Autodesk Inventor part; units mm, degrees
(part 10 of 12)
  line L8077 (-17.2005, 26.4334) -> (-16.2005, 26.4334)
  line L8078 (-16.2005, 26.4334) -> (-16.2005, 25.4334)
  line L8079 (-16.7593, 25.4334) -> (-17.7593, 25.4334)
  line L8080 (-17.7593, 25.4334) -> (-17.7593, 26.4334)
  line L8081 (-17.7593, 26.4334) -> (-16.7593, 26.4334)
  line L8082 (-16.7593, 26.4334) -> (-16.7593, 25.4334)
  line L8083 (-17.4197, 25.4334) -> (-18.4197, 25.4334)
  line L8084 (-18.4197, 25.4334) -> (-18.4197, 26.4334)
  line L8085 (-18.4197, 26.4334) -> (-17.4197, 26.4334)
  line L8086 (-17.4197, 26.4334) -> (-17.4197, 25.4334)
  line L8087 (-18.0166, 25.4334) -> (-19.0166, 25.4334)
  line L8088 (-19.0166, 25.4334) -> (-19.0166, 26.4334)
  line L8089 (-19.0166, 26.4334) -> (-18.0166, 26.4334)
  line L8090 (-18.0166, 26.4334) -> (-18.0166, 25.4334)
  line L8091 (-18.6643, 25.4334) -> (-19.6643, 25.4334)
  line L8092 (-19.6643, 25.4334) -> (-19.6643, 26.4334)
  line L8093 (-19.6643, 26.4334) -> (-18.6643, 26.4334)
  line L8094 (-18.6643, 26.4334) -> (-18.6643, 25.4334)
  line L8095 (-19.2739, 25.4334) -> (-20.2739, 25.4334)
  line L8096 (-20.2739, 25.4334) -> (-20.2739, 26.4334)
  line L8097 (-20.2739, 26.4334) -> (-19.2739, 26.4334)
  line L8098 (-19.2739, 26.4334) -> (-19.2739, 25.4334)
  line L8099 (-19.6676, 25.4334) -> (-20.6676, 25.4334)
  line L8100 (-20.6676, 25.4334) -> (-20.6676, 26.4334)
  line L8101 (-20.6676, 26.4334) -> (-19.6676, 26.4334)
  line L8102 (-19.6676, 26.4334) -> (-19.6676, 25.4334)
  line L8103 (-20.0867, 25.4334) -> (-21.0867, 25.4334)
  line L8104 (-21.0867, 25.4334) -> (-21.0867, 26.4334)
  line L8105 (-21.0867, 26.4334) -> (-20.0867, 26.4334)
  line L8106 (-20.0867, 26.4334) -> (-20.0867, 25.4334)
  line L8107 (-20.4931, 25.4334) -> (-21.4931, 25.4334)
  line L8108 (-21.4931, 25.4334) -> (-21.4931, 26.4334)
  line L8109 (-21.4931, 26.4334) -> (-20.4931, 26.4334)
  line L8110 (-20.4931, 26.4334) -> (-20.4931, 25.4334)
  line L8111 (-21.1916, 25.4334) -> (-22.1916, 25.4334)
  line L8112 (-22.1916, 25.4334) -> (-22.1916, 26.4334)
  line L8113 (-22.1916, 26.4334) -> (-21.1916, 26.4334)
  line L8114 (-21.1916, 26.4334) -> (-21.1916, 25.4334)
  line L8115 (-21.8393, 25.4334) -> (-22.8393, 25.4334)
  line L8116 (-22.8393, 25.4334) -> (-22.8393, 26.4334)
  line L8117 (-22.8393, 26.4334) -> (-21.8393, 26.4334)
  line L8118 (-21.8393, 26.4334) -> (-21.8393, 25.4334)
  line L8119 (-13.0255, 25.4588) -> (-14.0255, 25.4588)
  line L8120 (-14.0255, 25.4588) -> (-14.0255, 26.4588)
  line L8121 (-14.0255, 26.4588) -> (-13.0255, 26.4588)
  line L8122 (-13.0255, 26.4588) -> (-13.0255, 25.4588)
  line L8123 (-14.74, 25.4588) -> (-15.74, 25.4588)
  line L8124 (-15.74, 25.4588) -> (-15.74, 26.4588)
  line L8125 (-15.74, 26.4588) -> (-14.74, 26.4588)
  line L8126 (-14.74, 26.4588) -> (-14.74, 25.4588)
  line L8127 (-15.5147, 25.4588) -> (-16.5147, 25.4588)
  line L8128 (-16.5147, 25.4588) -> (-16.5147, 26.4588)
  line L8129 (-16.5147, 26.4588) -> (-15.5147, 26.4588)
  line L8130 (-15.5147, 26.4588) -> (-15.5147, 25.4588)
  line L8131 (-16.1878, 25.4588) -> (-17.1878, 25.4588)
  line L8132 (-17.1878, 25.4588) -> (-17.1878, 26.4588)
  line L8133 (-17.1878, 26.4588) -> (-16.1878, 26.4588)
  line L8134 (-16.1878, 26.4588) -> (-16.1878, 25.4588)
  line L8135 (-16.7847, 25.4588) -> (-17.7847, 25.4588)
  line L8136 (-17.7847, 25.4588) -> (-17.7847, 26.4588)
  line L8137 (-17.7847, 26.4588) -> (-16.7847, 26.4588)
  line L8138 (-16.7847, 26.4588) -> (-16.7847, 25.4588)
  line L8139 (-17.4197, 25.4588) -> (-18.4197, 25.4588)
  line L8140 (-18.4197, 25.4588) -> (-18.4197, 26.4588)
  line L8141 (-18.4197, 26.4588) -> (-17.4197, 26.4588)
  line L8142 (-17.4197, 26.4588) -> (-17.4197, 25.4588)
  line L8143 (-18.3341, 25.4588) -> (-19.3341, 25.4588)
  line L8144 (-19.3341, 25.4588) -> (-19.3341, 26.4588)
  line L8145 (-19.3341, 26.4588) -> (-18.3341, 26.4588)
  line L8146 (-18.3341, 26.4588) -> (-18.3341, 25.4588)
  line L8147 (-19.2739, 25.4588) -> (-20.2739, 25.4588)
  line L8148 (-20.2739, 25.4588) -> (-20.2739, 26.4588)
  line L8149 (-20.2739, 26.4588) -> (-19.2739, 26.4588)
  line L8150 (-19.2739, 26.4588) -> (-19.2739, 25.4588)
  line L8151 (-19.6676, 25.4588) -> (-20.6676, 25.4588)
  line L8152 (-20.6676, 25.4588) -> (-20.6676, 26.4588)
  line L8153 (-20.6676, 26.4588) -> (-19.6676, 26.4588)
  line L8154 (-19.6676, 26.4588) -> (-19.6676, 25.4588)
  line L8155 (-20.0867, 25.4588) -> (-21.0867, 25.4588)
  line L8156 (-21.0867, 25.4588) -> (-21.0867, 26.4588)
  line L8157 (-21.0867, 26.4588) -> (-20.0867, 26.4588)
  line L8158 (-20.0867, 26.4588) -> (-20.0867, 25.4588)
  line L8159 (-20.4931, 25.4588) -> (-21.4931, 25.4588)
  line L8160 (-21.4931, 25.4588) -> (-21.4931, 26.4588)
  line L8161 (-21.4931, 26.4588) -> (-20.4931, 26.4588)
  line L8162 (-20.4931, 26.4588) -> (-20.4931, 25.4588)
  line L8163 (-21.1916, 25.4588) -> (-22.1916, 25.4588)
  line L8164 (-22.1916, 25.4588) -> (-22.1916, 26.4588)
  line L8165 (-22.1916, 26.4588) -> (-21.1916, 26.4588)
  line L8166 (-21.1916, 26.4588) -> (-21.1916, 25.4588)
  line L8167 (-21.852, 25.4588) -> (-22.852, 25.4588)
  line L8168 (-22.852, 25.4588) -> (-22.852, 26.4588)
  line L8169 (-22.852, 26.4588) -> (-21.852, 26.4588)
  line L8170 (-21.852, 26.4588) -> (-21.852, 25.4588)
  line L8171 (-12.4667, 25.4842) -> (-13.4667, 25.4842)
  line L8172 (-13.4667, 25.4842) -> (-13.4667, 26.4842)
  line L8173 (-13.4667, 26.4842) -> (-12.4667, 26.4842)
  line L8174 (-12.4667, 26.4842) -> (-12.4667, 25.4842)
  line L8175 (-13.0509, 25.4842) -> (-14.0509, 25.4842)
  line L8176 (-14.0509, 25.4842) -> (-14.0509, 26.4842)
  line L8177 (-14.0509, 26.4842) -> (-13.0509, 26.4842)
  line L8178 (-13.0509, 26.4842) -> (-13.0509, 25.4842)
  line L8179 (-14.7654, 25.4842) -> (-15.7654, 25.4842)
  line L8180 (-15.7654, 25.4842) -> (-15.7654, 26.4842)
  line L8181 (-15.7654, 26.4842) -> (-14.7654, 26.4842)
  line L8182 (-14.7654, 26.4842) -> (-14.7654, 25.4842)
  line L8183 (-15.5528, 25.4842) -> (-16.5528, 25.4842)
  line L8184 (-16.5528, 25.4842) -> (-16.5528, 26.4842)
  line L8185 (-16.5528, 26.4842) -> (-15.5528, 26.4842)
  line L8186 (-15.5528, 26.4842) -> (-15.5528, 25.4842)
  line L8187 (-16.1497, 25.4842) -> (-17.1497, 25.4842)
  line L8188 (-17.1497, 25.4842) -> (-17.1497, 26.4842)
  line L8189 (-17.1497, 26.4842) -> (-16.1497, 26.4842)
  line L8190 (-16.1497, 26.4842) -> (-16.1497, 25.4842)
  line L8191 (-16.7974, 25.4842) -> (-17.7974, 25.4842)
  line L8192 (-17.7974, 25.4842) -> (-17.7974, 26.4842)
  line L8193 (-17.7974, 26.4842) -> (-16.7974, 26.4842)
  line L8194 (-16.7974, 26.4842) -> (-16.7974, 25.4842)
  line L8195 (-17.3943, 25.4842) -> (-18.3943, 25.4842)
  line L8196 (-18.3943, 25.4842) -> (-18.3943, 26.4842)
  line L8197 (-18.3943, 26.4842) -> (-17.3943, 26.4842)
  line L8198 (-17.3943, 26.4842) -> (-17.3943, 25.4842)
  line L8199 (-18.3341, 25.4842) -> (-19.3341, 25.4842)
  line L8200 (-19.3341, 25.4842) -> (-19.3341, 26.4842)
  line L8201 (-19.3341, 26.4842) -> (-18.3341, 26.4842)
  line L8202 (-18.3341, 26.4842) -> (-18.3341, 25.4842)
  line L8203 (-19.2739, 25.4842) -> (-20.2739, 25.4842)
  line L8204 (-20.2739, 25.4842) -> (-20.2739, 26.4842)
  line L8205 (-20.2739, 26.4842) -> (-19.2739, 26.4842)
  line L8206 (-19.2739, 26.4842) -> (-19.2739, 25.4842)
  line L8207 (-19.6676, 25.4842) -> (-20.6676, 25.4842)
  line L8208 (-20.6676, 25.4842) -> (-20.6676, 26.4842)
  line L8209 (-20.6676, 26.4842) -> (-19.6676, 26.4842)
  line L8210 (-19.6676, 26.4842) -> (-19.6676, 25.4842)
  line L8211 (-20.1121, 25.4842) -> (-21.1121, 25.4842)
  line L8212 (-21.1121, 25.4842) -> (-21.1121, 26.4842)
  line L8213 (-21.1121, 26.4842) -> (-20.1121, 26.4842)
  line L8214 (-20.1121, 26.4842) -> (-20.1121, 25.4842)
  line L8215 (-20.4931, 25.4842) -> (-21.4931, 25.4842)
  line L8216 (-21.4931, 25.4842) -> (-21.4931, 26.4842)
  line L8217 (-21.4931, 26.4842) -> (-20.4931, 26.4842)
  line L8218 (-20.4931, 26.4842) -> (-20.4931, 25.4842)
  line L8219 (-21.1789, 25.4842) -> (-22.1789, 25.4842)
  line L8220 (-22.1789, 25.4842) -> (-22.1789, 26.4842)
  line L8221 (-22.1789, 26.4842) -> (-21.1789, 26.4842)
  line L8222 (-21.1789, 26.4842) -> (-21.1789, 25.4842)
  line L8223 (-21.8647, 25.4842) -> (-22.8647, 25.4842)
  line L8224 (-22.8647, 25.4842) -> (-22.8647, 26.4842)
  line L8225 (-22.8647, 26.4842) -> (-21.8647, 26.4842)
  line L8226 (-21.8647, 26.4842) -> (-21.8647, 25.4842)
  line L8227 (-12.4921, 25.5096) -> (-13.4921, 25.5096)
  line L8228 (-13.4921, 25.5096) -> (-13.4921, 26.5096)
  line L8229 (-13.4921, 26.5096) -> (-12.4921, 26.5096)
  line L8230 (-12.4921, 26.5096) -> (-12.4921, 25.5096)
  line L8231 (-13.0763, 25.5096) -> (-14.0763, 25.5096)
  line L8232 (-14.0763, 25.5096) -> (-14.0763, 26.5096)
  line L8233 (-14.0763, 26.5096) -> (-13.0763, 26.5096)
  line L8234 (-13.0763, 26.5096) -> (-13.0763, 25.5096)
  line L8235 (-14.7908, 25.5096) -> (-15.7908, 25.5096)
  line L8236 (-15.7908, 25.5096) -> (-15.7908, 26.5096)
  line L8237 (-15.7908, 26.5096) -> (-14.7908, 26.5096)
  line L8238 (-14.7908, 26.5096) -> (-14.7908, 25.5096)
  line L8239 (-15.8576, 25.5096) -> (-16.8576, 25.5096)
  line L8240 (-16.8576, 25.5096) -> (-16.8576, 26.5096)
  line L8241 (-16.8576, 26.5096) -> (-15.8576, 26.5096)
  line L8242 (-15.8576, 26.5096) -> (-15.8576, 25.5096)
  line L8243 (-16.8228, 25.5096) -> (-17.8228, 25.5096)
  line L8244 (-17.8228, 25.5096) -> (-17.8228, 26.5096)
  line L8245 (-17.8228, 26.5096) -> (-16.8228, 26.5096)
  line L8246 (-16.8228, 26.5096) -> (-16.8228, 25.5096)
  line L8247 (-17.3943, 25.5096) -> (-18.3943, 25.5096)
  line L8248 (-18.3943, 25.5096) -> (-18.3943, 26.5096)
  line L8249 (-18.3943, 26.5096) -> (-17.3943, 26.5096)
  line L8250 (-17.3943, 26.5096) -> (-17.3943, 25.5096)
  line L8251 (-18.3341, 25.5096) -> (-19.3341, 25.5096)
  line L8252 (-19.3341, 25.5096) -> (-19.3341, 26.5096)
  line L8253 (-19.3341, 26.5096) -> (-18.3341, 26.5096)
  line L8254 (-18.3341, 26.5096) -> (-18.3341, 25.5096)
  line L8255 (-19.2739, 25.5096) -> (-20.2739, 25.5096)
  line L8256 (-20.2739, 25.5096) -> (-20.2739, 26.5096)
  line L8257 (-20.2739, 26.5096) -> (-19.2739, 26.5096)
  line L8258 (-19.2739, 26.5096) -> (-19.2739, 25.5096)
  line L8259 (-19.6676, 25.5096) -> (-20.6676, 25.5096)
  line L8260 (-20.6676, 25.5096) -> (-20.6676, 26.5096)
  line L8261 (-20.6676, 26.5096) -> (-19.6676, 26.5096)
  line L8262 (-19.6676, 26.5096) -> (-19.6676, 25.5096)
  line L8263 (-20.1121, 25.5096) -> (-21.1121, 25.5096)
  line L8264 (-21.1121, 25.5096) -> (-21.1121, 26.5096)
  line L8265 (-21.1121, 26.5096) -> (-20.1121, 26.5096)
  line L8266 (-20.1121, 26.5096) -> (-20.1121, 25.5096)
  line L8267 (-20.4931, 25.5096) -> (-21.4931, 25.5096)
  line L8268 (-21.4931, 25.5096) -> (-21.4931, 26.5096)
  line L8269 (-21.4931, 26.5096) -> (-20.4931, 26.5096)
  line L8270 (-20.4931, 26.5096) -> (-20.4931, 25.5096)
  line L8271 (-21.1789, 25.5096) -> (-22.1789, 25.5096)
  line L8272 (-22.1789, 25.5096) -> (-22.1789, 26.5096)
  line L8273 (-22.1789, 26.5096) -> (-21.1789, 26.5096)
  line L8274 (-21.1789, 26.5096) -> (-21.1789, 25.5096)
  line L8275 (-21.8774, 25.5096) -> (-22.8774, 25.5096)
  line L8276 (-22.8774, 25.5096) -> (-22.8774, 26.5096)
  line L8277 (-22.8774, 26.5096) -> (-21.8774, 26.5096)
  line L8278 (-21.8774, 26.5096) -> (-21.8774, 25.5096)
  line L8279 (-12.5175, 25.535) -> (-13.5175, 25.535)
  line L8280 (-13.5175, 25.535) -> (-13.5175, 26.535)
  line L8281 (-13.5175, 26.535) -> (-12.5175, 26.535)
  line L8282 (-12.5175, 26.535) -> (-12.5175, 25.535)
  line L8283 (-13.1017, 25.535) -> (-14.1017, 25.535)
  line L8284 (-14.1017, 25.535) -> (-14.1017, 26.535)
  line L8285 (-14.1017, 26.535) -> (-13.1017, 26.535)
  line L8286 (-13.1017, 26.535) -> (-13.1017, 25.535)
  line L8287 (-14.8162, 25.535) -> (-15.8162, 25.535)
  line L8288 (-15.8162, 25.535) -> (-15.8162, 26.535)
  line L8289 (-15.8162, 26.535) -> (-14.8162, 26.535)
  line L8290 (-14.8162, 26.535) -> (-14.8162, 25.535)
  line L8291 (-15.8449, 25.535) -> (-16.8449, 25.535)
  line L8292 (-16.8449, 25.535) -> (-16.8449, 26.535)
  line L8293 (-16.8449, 26.535) -> (-15.8449, 26.535)
  line L8294 (-15.8449, 26.535) -> (-15.8449, 25.535)
  line L8295 (-16.8482, 25.535) -> (-17.8482, 25.535)
  line L8296 (-17.8482, 25.535) -> (-17.8482, 26.535)
  line L8297 (-17.8482, 26.535) -> (-16.8482, 26.535)
  line L8298 (-16.8482, 26.535) -> (-16.8482, 25.535)
  line L8299 (-17.3689, 25.535) -> (-18.3689, 25.535)
  line L8300 (-18.3689, 25.535) -> (-18.3689, 26.535)
  line L8301 (-18.3689, 26.535) -> (-17.3689, 26.535)
  line L8302 (-17.3689, 26.535) -> (-17.3689, 25.535)
  line L8303 (-18.3214, 25.535) -> (-19.3214, 25.535)
  line L8304 (-19.3214, 25.535) -> (-19.3214, 26.535)
  line L8305 (-19.3214, 26.535) -> (-18.3214, 26.535)
  line L8306 (-18.3214, 26.535) -> (-18.3214, 25.535)
  line L8307 (-19.2739, 25.535) -> (-20.2739, 25.535)
  line L8308 (-20.2739, 25.535) -> (-20.2739, 26.535)
  line L8309 (-20.2739, 26.535) -> (-19.2739, 26.535)
  line L8310 (-19.2739, 26.535) -> (-19.2739, 25.535)
  line L8311 (-19.6549, 25.535) -> (-20.6549, 25.535)
  line L8312 (-20.6549, 25.535) -> (-20.6549, 26.535)
  line L8313 (-20.6549, 26.535) -> (-19.6549, 26.535)
  line L8314 (-19.6549, 26.535) -> (-19.6549, 25.535)
  line L8315 (-20.1121, 25.535) -> (-21.1121, 25.535)
  line L8316 (-21.1121, 25.535) -> (-21.1121, 26.535)
  line L8317 (-21.1121, 26.535) -> (-20.1121, 26.535)
  line L8318 (-20.1121, 26.535) -> (-20.1121, 25.535)
  line L8319 (-20.4931, 25.535) -> (-21.4931, 25.535)
  line L8320 (-21.4931, 25.535) -> (-21.4931, 26.535)
  line L8321 (-21.4931, 26.535) -> (-20.4931, 26.535)
  line L8322 (-20.4931, 26.535) -> (-20.4931, 25.535)
  line L8323 (-21.1662, 25.535) -> (-22.1662, 25.535)
  line L8324 (-22.1662, 25.535) -> (-22.1662, 26.535)
  line L8325 (-22.1662, 26.535) -> (-21.1662, 26.535)
  line L8326 (-21.1662, 26.535) -> (-21.1662, 25.535)
  line L8327 (-21.8901, 25.535) -> (-22.8901, 25.535)
  line L8328 (-22.8901, 25.535) -> (-22.8901, 26.535)
  line L8329 (-22.8901, 26.535) -> (-21.8901, 26.535)
  line L8330 (-21.8901, 26.535) -> (-21.8901, 25.535)
  line L8331 (-12.5302, 25.5604) -> (-13.5302, 25.5604)
  line L8332 (-13.5302, 25.5604) -> (-13.5302, 26.5604)
  line L8333 (-13.5302, 26.5604) -> (-12.5302, 26.5604)
  line L8334 (-12.5302, 26.5604) -> (-12.5302, 25.5604)
  line L8335 (-13.1144, 25.5604) -> (-14.1144, 25.5604)
  line L8336 (-14.1144, 25.5604) -> (-14.1144, 26.5604)
  line L8337 (-14.1144, 26.5604) -> (-13.1144, 26.5604)
  line L8338 (-13.1144, 26.5604) -> (-13.1144, 25.5604)
  line L8339 (-14.7447, 26.0477) -> (-14.7701, 26.0477)
  line L8340 (-14.7701, 26.0477) -> (-14.7701, 26.0731)
  line L8341 (-14.7701, 26.0731) -> (-14.7447, 26.0731)
  line L8342 (-14.7447, 26.0731) -> (-14.7447, 26.0477)
  line L8343 (-14.8289, 25.5604) -> (-15.8289, 25.5604)
  line L8344 (-15.8289, 25.5604) -> (-15.8289, 26.5604)
  line L8345 (-15.8289, 26.5604) -> (-14.8289, 26.5604)
  line L8346 (-14.8289, 26.5604) -> (-14.8289, 25.5604)
  line L8347 (-15.8449, 25.5604) -> (-16.8449, 25.5604)
  line L8348 (-16.8449, 25.5604) -> (-16.8449, 26.5604)
  line L8349 (-16.8449, 26.5604) -> (-15.8449, 26.5604)
  line L8350 (-15.8449, 26.5604) -> (-15.8449, 25.5604)
  line L8351 (-17.1022, 25.5604) -> (-18.1022, 25.5604)
  line L8352 (-18.1022, 25.5604) -> (-18.1022, 26.5604)
  line L8353 (-18.1022, 26.5604) -> (-17.1022, 26.5604)
  line L8354 (-17.1022, 26.5604) -> (-17.1022, 25.5604)
  line L8355 (-18.3214, 25.5604) -> (-19.3214, 25.5604)
  line L8356 (-19.3214, 25.5604) -> (-19.3214, 26.5604)
  line L8357 (-19.3214, 26.5604) -> (-18.3214, 26.5604)
  line L8358 (-18.3214, 26.5604) -> (-18.3214, 25.5604)
  line L8359 (-19.2993, 25.5604) -> (-20.2993, 25.5604)
  line L8360 (-20.2993, 25.5604) -> (-20.2993, 26.5604)
  line L8361 (-20.2993, 26.5604) -> (-19.2993, 26.5604)
  line L8362 (-19.2993, 26.5604) -> (-19.2993, 25.5604)
  line L8363 (-19.6422, 25.5604) -> (-20.6422, 25.5604)
  line L8364 (-20.6422, 25.5604) -> (-20.6422, 26.5604)
  line L8365 (-20.6422, 26.5604) -> (-19.6422, 26.5604)
  line L8366 (-19.6422, 26.5604) -> (-19.6422, 25.5604)
  line L8367 (-20.1375, 25.5604) -> (-21.1375, 25.5604)
  line L8368 (-21.1375, 25.5604) -> (-21.1375, 26.5604)
  line L8369 (-21.1375, 26.5604) -> (-20.1375, 26.5604)
  line L8370 (-20.1375, 26.5604) -> (-20.1375, 25.5604)
  line L8371 (-20.5058, 25.5604) -> (-21.5058, 25.5604)
  line L8372 (-21.5058, 25.5604) -> (-21.5058, 26.5604)
  line L8373 (-21.5058, 26.5604) -> (-20.5058, 26.5604)
  line L8374 (-20.5058, 26.5604) -> (-20.5058, 25.5604)
  line L8375 (-21.1535, 25.5604) -> (-22.1535, 25.5604)
  line L8376 (-22.1535, 25.5604) -> (-22.1535, 26.5604)
  line L8377 (-22.1535, 26.5604) -> (-21.1535, 26.5604)
  line L8378 (-21.1535, 26.5604) -> (-21.1535, 25.5604)
  line L8379 (-21.9028, 25.5604) -> (-22.9028, 25.5604)
  line L8380 (-22.9028, 25.5604) -> (-22.9028, 26.5604)
  line L8381 (-22.9028, 26.5604) -> (-21.9028, 26.5604)
  line L8382 (-21.9028, 26.5604) -> (-21.9028, 25.5604)
  line L8383 (-12.5556, 25.5858) -> (-13.5556, 25.5858)
  line L8384 (-13.5556, 25.5858) -> (-13.5556, 26.5858)
  line L8385 (-13.5556, 26.5858) -> (-12.5556, 26.5858)
  line L8386 (-12.5556, 26.5858) -> (-12.5556, 25.5858)
  line L8387 (-13.1398, 25.5858) -> (-14.1398, 25.5858)
  line L8388 (-14.1398, 25.5858) -> (-14.1398, 26.5858)
  line L8389 (-14.1398, 26.5858) -> (-13.1398, 26.5858)
  line L8390 (-13.1398, 26.5858) -> (-13.1398, 25.5858)
  line L8391 (-14.2701, 25.5858) -> (-15.2701, 25.5858)
  line L8392 (-15.2701, 25.5858) -> (-15.2701, 26.5858)
  line L8393 (-15.2701, 26.5858) -> (-14.2701, 26.5858)
  line L8394 (-14.2701, 26.5858) -> (-14.2701, 25.5858)
  line L8395 (-14.867, 25.5858) -> (-15.867, 25.5858)
  line L8396 (-15.867, 25.5858) -> (-15.867, 26.5858)
  line L8397 (-15.867, 26.5858) -> (-14.867, 26.5858)
  line L8398 (-14.867, 26.5858) -> (-14.867, 25.5858)
  line L8399 (-15.8322, 25.5858) -> (-16.8322, 25.5858)
  line L8400 (-16.8322, 25.5858) -> (-16.8322, 26.5858)
  line L8401 (-16.8322, 26.5858) -> (-15.8322, 26.5858)
  line L8402 (-15.8322, 26.5858) -> (-15.8322, 25.5858)
  line L8403 (-17.1149, 25.5858) -> (-18.1149, 25.5858)
  line L8404 (-18.1149, 25.5858) -> (-18.1149, 26.5858)
  line L8405 (-18.1149, 26.5858) -> (-17.1149, 26.5858)
  line L8406 (-17.1149, 26.5858) -> (-17.1149, 25.5858)
  line L8407 (-18.3214, 25.5858) -> (-19.3214, 25.5858)
  line L8408 (-19.3214, 25.5858) -> (-19.3214, 26.5858)
  line L8409 (-19.3214, 26.5858) -> (-18.3214, 26.5858)
  line L8410 (-18.3214, 26.5858) -> (-18.3214, 25.5858)
  line L8411 (-19.2993, 25.5858) -> (-20.2993, 25.5858)
  line L8412 (-20.2993, 25.5858) -> (-20.2993, 26.5858)
  line L8413 (-20.2993, 26.5858) -> (-19.2993, 26.5858)
  line L8414 (-19.2993, 26.5858) -> (-19.2993, 25.5858)
  line L8415 (-19.6422, 25.5858) -> (-20.6422, 25.5858)
  line L8416 (-20.6422, 25.5858) -> (-20.6422, 26.5858)
  line L8417 (-20.6422, 26.5858) -> (-19.6422, 26.5858)
  line L8418 (-19.6422, 26.5858) -> (-19.6422, 25.5858)
  line L8419 (-20.1375, 25.5858) -> (-21.1375, 25.5858)
  line L8420 (-21.1375, 25.5858) -> (-21.1375, 26.5858)
  line L8421 (-21.1375, 26.5858) -> (-20.1375, 26.5858)
  line L8422 (-20.1375, 26.5858) -> (-20.1375, 25.5858)
  line L8423 (-20.5058, 25.5858) -> (-21.5058, 25.5858)
  line L8424 (-21.5058, 25.5858) -> (-21.5058, 26.5858)
  line L8425 (-21.5058, 26.5858) -> (-20.5058, 26.5858)
  line L8426 (-20.5058, 26.5858) -> (-20.5058, 25.5858)
  line L8427 (-21.1535, 25.5858) -> (-22.1535, 25.5858)
  line L8428 (-22.1535, 25.5858) -> (-22.1535, 26.5858)
  line L8429 (-22.1535, 26.5858) -> (-21.1535, 26.5858)
  line L8430 (-21.1535, 26.5858) -> (-21.1535, 25.5858)
  line L8431 (-21.9155, 25.5858) -> (-22.9155, 25.5858)
  line L8432 (-22.9155, 25.5858) -> (-22.9155, 26.5858)
  line L8433 (-22.9155, 26.5858) -> (-21.9155, 26.5858)
  line L8434 (-21.9155, 26.5858) -> (-21.9155, 25.5858)
  line L8435 (-12.581, 25.6112) -> (-13.581, 25.6112)
  line L8436 (-13.581, 25.6112) -> (-13.581, 26.6112)
  line L8437 (-13.581, 26.6112) -> (-12.581, 26.6112)
  line L8438 (-12.581, 26.6112) -> (-12.581, 25.6112)
  line L8439 (-13.1652, 25.6112) -> (-14.1652, 25.6112)
  line L8440 (-14.1652, 25.6112) -> (-14.1652, 26.6112)
  line L8441 (-14.1652, 26.6112) -> (-13.1652, 26.6112)
  line L8442 (-13.1652, 26.6112) -> (-13.1652, 25.6112)
  line L8443 (-14.2955, 25.6112) -> (-15.2955, 25.6112)
  line L8444 (-15.2955, 25.6112) -> (-15.2955, 26.6112)
  line L8445 (-15.2955, 26.6112) -> (-14.2955, 26.6112)
  line L8446 (-14.2955, 26.6112) -> (-14.2955, 25.6112)
  line L8447 (-14.8924, 25.6112) -> (-15.8924, 25.6112)
  line L8448 (-15.8924, 25.6112) -> (-15.8924, 26.6112)
  line L8449 (-15.8924, 26.6112) -> (-14.8924, 26.6112)
  line L8450 (-14.8924, 26.6112) -> (-14.8924, 25.6112)
  line L8451 (-15.8195, 25.6112) -> (-16.8195, 25.6112)
  line L8452 (-16.8195, 25.6112) -> (-16.8195, 26.6112)
  line L8453 (-16.8195, 26.6112) -> (-15.8195, 26.6112)
  line L8454 (-15.8195, 26.6112) -> (-15.8195, 25.6112)
  line L8455 (-17.1022, 25.6112) -> (-18.1022, 25.6112)
  line L8456 (-18.1022, 25.6112) -> (-18.1022, 26.6112)
  line L8457 (-18.1022, 26.6112) -> (-17.1022, 26.6112)
  line L8458 (-17.1022, 26.6112) -> (-17.1022, 25.6112)
  line L8459 (-18.3087, 25.6112) -> (-19.3087, 25.6112)
  line L8460 (-19.3087, 25.6112) -> (-19.3087, 26.6112)
  line L8461 (-19.3087, 26.6112) -> (-18.3087, 26.6112)
  line L8462 (-18.3087, 26.6112) -> (-18.3087, 25.6112)
  line L8463 (-19.2993, 25.6112) -> (-20.2993, 25.6112)
  line L8464 (-20.2993, 25.6112) -> (-20.2993, 26.6112)
  line L8465 (-20.2993, 26.6112) -> (-19.2993, 26.6112)
  line L8466 (-19.2993, 26.6112) -> (-19.2993, 25.6112)
  line L8467 (-19.6422, 25.6112) -> (-20.6422, 25.6112)
  line L8468 (-20.6422, 25.6112) -> (-20.6422, 26.6112)
  line L8469 (-20.6422, 26.6112) -> (-19.6422, 26.6112)
  line L8470 (-19.6422, 26.6112) -> (-19.6422, 25.6112)
  line L8471 (-20.1375, 25.6112) -> (-21.1375, 25.6112)
  line L8472 (-21.1375, 25.6112) -> (-21.1375, 26.6112)
  line L8473 (-21.1375, 26.6112) -> (-20.1375, 26.6112)
  line L8474 (-20.1375, 26.6112) -> (-20.1375, 25.6112)
  line L8475 (-20.5058, 25.6112) -> (-21.5058, 25.6112)
  line L8476 (-21.5058, 25.6112) -> (-21.5058, 26.6112)
  line L8477 (-21.5058, 26.6112) -> (-20.5058, 26.6112)
  line L8478 (-20.5058, 26.6112) -> (-20.5058, 25.6112)
  line L8479 (-21.1408, 25.6112) -> (-22.1408, 25.6112)
  line L8480 (-22.1408, 25.6112) -> (-22.1408, 26.6112)
  line L8481 (-22.1408, 26.6112) -> (-21.1408, 26.6112)
  line L8482 (-21.1408, 26.6112) -> (-21.1408, 25.6112)
  line L8483 (-21.9282, 25.6112) -> (-22.9282, 25.6112)
  line L8484 (-22.9282, 25.6112) -> (-22.9282, 26.6112)
  line L8485 (-22.9282, 26.6112) -> (-21.9282, 26.6112)
  line L8486 (-21.9282, 26.6112) -> (-21.9282, 25.6112)
  line L8487 (-12.5937, 25.6366) -> (-13.5937, 25.6366)
  line L8488 (-13.5937, 25.6366) -> (-13.5937, 26.6366)
  line L8489 (-13.5937, 26.6366) -> (-12.5937, 26.6366)
  line L8490 (-12.5937, 26.6366) -> (-12.5937, 25.6366)
  line L8491 (-13.1779, 25.6366) -> (-14.1779, 25.6366)
  line L8492 (-14.1779, 25.6366) -> (-14.1779, 26.6366)
  line L8493 (-14.1779, 26.6366) -> (-13.1779, 26.6366)
  line L8494 (-13.1779, 26.6366) -> (-13.1779, 25.6366)
  line L8495 (-14.3209, 25.6366) -> (-15.3209, 25.6366)
  line L8496 (-15.3209, 25.6366) -> (-15.3209, 26.6366)
  line L8497 (-15.3209, 26.6366) -> (-14.3209, 26.6366)
  line L8498 (-14.3209, 26.6366) -> (-14.3209, 25.6366)
  line L8499 (-14.9178, 25.6366) -> (-15.9178, 25.6366)
  line L8500 (-15.9178, 25.6366) -> (-15.9178, 26.6366)
  line L8501 (-15.9178, 26.6366) -> (-14.9178, 26.6366)
  line L8502 (-14.9178, 26.6366) -> (-14.9178, 25.6366)
  line L8503 (-15.8068, 25.6366) -> (-16.8068, 25.6366)
  line L8504 (-16.8068, 25.6366) -> (-16.8068, 26.6366)
  line L8505 (-16.8068, 26.6366) -> (-15.8068, 26.6366)
  line L8506 (-15.8068, 26.6366) -> (-15.8068, 25.6366)
  line L8507 (-17.1022, 25.6366) -> (-18.1022, 25.6366)
  line L8508 (-18.1022, 25.6366) -> (-18.1022, 26.6366)
  line L8509 (-18.1022, 26.6366) -> (-17.1022, 26.6366)
  line L8510 (-17.1022, 26.6366) -> (-17.1022, 25.6366)
  line L8511 (-17.9658, 25.6366) -> (-18.9658, 25.6366)
  line L8512 (-18.9658, 25.6366) -> (-18.9658, 26.6366)
  line L8513 (-18.9658, 26.6366) -> (-17.9658, 26.6366)
  line L8514 (-17.9658, 26.6366) -> (-17.9658, 25.6366)
  line L8515 (-18.5119, 25.6366) -> (-19.5119, 25.6366)
  line L8516 (-19.5119, 25.6366) -> (-19.5119, 26.6366)
  line L8517 (-19.5119, 26.6366) -> (-18.5119, 26.6366)
  line L8518 (-18.5119, 26.6366) -> (-18.5119, 25.6366)
  line L8519 (-19.2993, 25.6366) -> (-20.2993, 25.6366)
  line L8520 (-20.2993, 25.6366) -> (-20.2993, 26.6366)
  line L8521 (-20.2993, 26.6366) -> (-19.2993, 26.6366)
  line L8522 (-19.2993, 26.6366) -> (-19.2993, 25.6366)
  line L8523 (-19.6422, 25.6366) -> (-20.6422, 25.6366)
  line L8524 (-20.6422, 25.6366) -> (-20.6422, 26.6366)
  line L8525 (-20.6422, 26.6366) -> (-19.6422, 26.6366)
  line L8526 (-19.6422, 26.6366) -> (-19.6422, 25.6366)
  line L8527 (-20.3407, 25.6366) -> (-21.3407, 25.6366)
  line L8528 (-21.3407, 25.6366) -> (-21.3407, 26.6366)
  line L8529 (-21.3407, 26.6366) -> (-20.3407, 26.6366)
  line L8530 (-20.3407, 26.6366) -> (-20.3407, 25.6366)
  line L8531 (-21.1281, 25.6366) -> (-22.1281, 25.6366)
  line L8532 (-22.1281, 25.6366) -> (-22.1281, 26.6366)
  line L8533 (-22.1281, 26.6366) -> (-21.1281, 26.6366)
  line L8534 (-21.1281, 26.6366) -> (-21.1281, 25.6366)
  line L8535 (-21.9409, 25.6366) -> (-22.9409, 25.6366)
  line L8536 (-22.9409, 25.6366) -> (-22.9409, 26.6366)
  line L8537 (-22.9409, 26.6366) -> (-21.9409, 26.6366)
  line L8538 (-21.9409, 26.6366) -> (-21.9409, 25.6366)
  line L8539 (-12.6191, 25.662) -> (-13.6191, 25.662)
  line L8540 (-13.6191, 25.662) -> (-13.6191, 26.662)
  line L8541 (-13.6191, 26.662) -> (-12.6191, 26.662)
  line L8542 (-12.6191, 26.662) -> (-12.6191, 25.662)
  line L8543 (-13.2033, 25.662) -> (-14.2033, 25.662)
  line L8544 (-14.2033, 25.662) -> (-14.2033, 26.662)
  line L8545 (-14.2033, 26.662) -> (-13.2033, 26.662)
  line L8546 (-13.2033, 26.662) -> (-13.2033, 25.662)
  line L8547 (-14.3336, 25.662) -> (-15.3336, 25.662)
  line L8548 (-15.3336, 25.662) -> (-15.3336, 26.662)
  line L8549 (-15.3336, 26.662) -> (-14.3336, 26.662)
  line L8550 (-14.3336, 26.662) -> (-14.3336, 25.662)
  line L8551 (-14.9305, 25.662) -> (-15.9305, 25.662)
  line L8552 (-15.9305, 25.662) -> (-15.9305, 26.662)
  line L8553 (-15.9305, 26.662) -> (-14.9305, 26.662)
  line L8554 (-14.9305, 26.662) -> (-14.9305, 25.662)
  line L8555 (-15.7941, 25.662) -> (-16.7941, 25.662)
  line L8556 (-16.7941, 25.662) -> (-16.7941, 26.662)
  line L8557 (-16.7941, 26.662) -> (-15.7941, 26.662)
  line L8558 (-15.7941, 26.662) -> (-15.7941, 25.662)
  line L8559 (-17.1149, 25.662) -> (-18.1149, 25.662)
  line L8560 (-18.1149, 25.662) -> (-18.1149, 26.662)
  line L8561 (-18.1149, 26.662) -> (-17.1149, 26.662)
  line L8562 (-17.1149, 26.662) -> (-17.1149, 25.662)
  line L8563 (-17.9658, 25.662) -> (-18.9658, 25.662)
  line L8564 (-18.9658, 25.662) -> (-18.9658, 26.662)
  line L8565 (-18.9658, 26.662) -> (-17.9658, 26.662)
  line L8566 (-17.9658, 26.662) -> (-17.9658, 25.662)
  line L8567 (-18.5119, 25.662) -> (-19.5119, 25.662)
  line L8568 (-19.5119, 25.662) -> (-19.5119, 26.662)
  line L8569 (-19.5119, 26.662) -> (-18.5119, 26.662)
  line L8570 (-18.5119, 26.662) -> (-18.5119, 25.662)
  line L8571 (-19.4644, 25.662) -> (-20.4644, 25.662)
  line L8572 (-20.4644, 25.662) -> (-20.4644, 26.662)
  line L8573 (-20.4644, 26.662) -> (-19.4644, 26.662)
  line L8574 (-19.4644, 26.662) -> (-19.4644, 25.662)
  line L8575 (-20.3407, 25.662) -> (-21.3407, 25.662)
  line L8576 (-21.3407, 25.662) -> (-21.3407, 26.662)
  line L8577 (-21.3407, 26.662) -> (-20.3407, 26.662)
  line L8578 (-20.3407, 26.662) -> (-20.3407, 25.662)
  line L8579 (-21.1281, 25.662) -> (-22.1281, 25.662)
  line L8580 (-22.1281, 25.662) -> (-22.1281, 26.662)
  line L8581 (-22.1281, 26.662) -> (-21.1281, 26.662)
  line L8582 (-21.1281, 26.662) -> (-21.1281, 25.662)
  line L8583 (-21.9536, 25.662) -> (-22.9536, 25.662)
  line L8584 (-22.9536, 25.662) -> (-22.9536, 26.662)
  line L8585 (-22.9536, 26.662) -> (-21.9536, 26.662)
  line L8586 (-21.9536, 26.662) -> (-21.9536, 25.662)
  line L8587 (-12.6445, 25.6874) -> (-13.6445, 25.6874)
  line L8588 (-13.6445, 25.6874) -> (-13.6445, 26.6874)
  line L8589 (-13.6445, 26.6874) -> (-12.6445, 26.6874)
  line L8590 (-12.6445, 26.6874) -> (-12.6445, 25.6874)
  line L8591 (-13.2287, 25.6874) -> (-14.2287, 25.6874)
  line L8592 (-14.2287, 25.6874) -> (-14.2287, 26.6874)
  line L8593 (-14.2287, 26.6874) -> (-13.2287, 26.6874)
  line L8594 (-13.2287, 26.6874) -> (-13.2287, 25.6874)
  line L8595 (-14.359, 25.6874) -> (-15.359, 25.6874)
  line L8596 (-15.359, 25.6874) -> (-15.359, 26.6874)
  line L8597 (-15.359, 26.6874) -> (-14.359, 26.6874)
  line L8598 (-14.359, 26.6874) -> (-14.359, 25.6874)
  line L8599 (-14.9559, 25.6874) -> (-15.9559, 25.6874)
  line L8600 (-15.9559, 25.6874) -> (-15.9559, 26.6874)
  line L8601 (-15.9559, 26.6874) -> (-14.9559, 26.6874)
  line L8602 (-14.9559, 26.6874) -> (-14.9559, 25.6874)
  line L8603 (-15.7814, 25.6874) -> (-16.7814, 25.6874)
  line L8604 (-16.7814, 25.6874) -> (-16.7814, 26.6874)
  line L8605 (-16.7814, 26.6874) -> (-15.7814, 26.6874)
  line L8606 (-15.7814, 26.6874) -> (-15.7814, 25.6874)
  line L8607 (-17.1022, 25.6874) -> (-18.1022, 25.6874)
  line L8608 (-18.1022, 25.6874) -> (-18.1022, 26.6874)
  line L8609 (-18.1022, 26.6874) -> (-17.1022, 26.6874)
  line L8610 (-17.1022, 26.6874) -> (-17.1022, 25.6874)
  line L8611 (-17.9658, 25.6874) -> (-18.9658, 25.6874)
  line L8612 (-18.9658, 25.6874) -> (-18.9658, 26.6874)
  line L8613 (-18.9658, 26.6874) -> (-17.9658, 26.6874)
  line L8614 (-17.9658, 26.6874) -> (-17.9658, 25.6874)
  line L8615 (-18.5119, 25.6874) -> (-19.5119, 25.6874)
  line L8616 (-19.5119, 25.6874) -> (-19.5119, 26.6874)
  line L8617 (-19.5119, 26.6874) -> (-18.5119, 26.6874)
  line L8618 (-18.5119, 26.6874) -> (-18.5119, 25.6874)
  line L8619 (-19.4644, 25.6874) -> (-20.4644, 25.6874)
  line L8620 (-20.4644, 25.6874) -> (-20.4644, 26.6874)
  line L8621 (-20.4644, 26.6874) -> (-19.4644, 26.6874)
  line L8622 (-19.4644, 26.6874) -> (-19.4644, 25.6874)
  line L8623 (-20.3407, 25.6874) -> (-21.3407, 25.6874)
  line L8624 (-21.3407, 25.6874) -> (-21.3407, 26.6874)
  line L8625 (-21.3407, 26.6874) -> (-20.3407, 26.6874)
  line L8626 (-20.3407, 26.6874) -> (-20.3407, 25.6874)
  line L8627 (-21.1154, 25.6874) -> (-22.1154, 25.6874)
  line L8628 (-22.1154, 25.6874) -> (-22.1154, 26.6874)
  line L8629 (-22.1154, 26.6874) -> (-21.1154, 26.6874)
  line L8630 (-21.1154, 26.6874) -> (-21.1154, 25.6874)
  line L8631 (-21.9663, 25.6874) -> (-22.9663, 25.6874)
  line L8632 (-22.9663, 25.6874) -> (-22.9663, 26.6874)
  line L8633 (-22.9663, 26.6874) -> (-21.9663, 26.6874)
  line L8634 (-21.9663, 26.6874) -> (-21.9663, 25.6874)
  line L8635 (-12.6699, 25.7128) -> (-13.6699, 25.7128)
  line L8636 (-13.6699, 25.7128) -> (-13.6699, 26.7128)
  line L8637 (-13.6699, 26.7128) -> (-12.6699, 26.7128)
  line L8638 (-12.6699, 26.7128) -> (-12.6699, 25.7128)
  line L8639 (-14.3844, 25.7128) -> (-15.3844, 25.7128)
  line L8640 (-15.3844, 25.7128) -> (-15.3844, 26.7128)
  line L8641 (-15.3844, 26.7128) -> (-14.3844, 26.7128)
  line L8642 (-14.3844, 26.7128) -> (-14.3844, 25.7128)
  line L8643 (-14.9813, 25.7128) -> (-15.9813, 25.7128)
  line L8644 (-15.9813, 25.7128) -> (-15.9813, 26.7128)
  line L8645 (-15.9813, 26.7128) -> (-14.9813, 26.7128)
  line L8646 (-14.9813, 26.7128) -> (-14.9813, 25.7128)
  line L8647 (-15.756, 25.7128) -> (-16.756, 25.7128)
  line L8648 (-16.756, 25.7128) -> (-16.756, 26.7128)
  line L8649 (-16.756, 26.7128) -> (-15.756, 26.7128)
  line L8650 (-15.756, 26.7128) -> (-15.756, 25.7128)
  line L8651 (-17.1022, 25.7128) -> (-18.1022, 25.7128)
  line L8652 (-18.1022, 25.7128) -> (-18.1022, 26.7128)
  line L8653 (-18.1022, 26.7128) -> (-17.1022, 26.7128)
  line L8654 (-17.1022, 26.7128) -> (-17.1022, 25.7128)
  line L8655 (-17.9658, 25.7128) -> (-18.9658, 25.7128)
  line L8656 (-18.9658, 25.7128) -> (-18.9658, 26.7128)
  line L8657 (-18.9658, 26.7128) -> (-17.9658, 26.7128)
  line L8658 (-17.9658, 26.7128) -> (-17.9658, 25.7128)
  line L8659 (-18.5119, 25.7128) -> (-19.5119, 25.7128)
  line L8660 (-19.5119, 25.7128) -> (-19.5119, 26.7128)
  line L8661 (-19.5119, 26.7128) -> (-18.5119, 26.7128)
  line L8662 (-18.5119, 26.7128) -> (-18.5119, 25.7128)
  line L8663 (-19.4644, 25.7128) -> (-20.4644, 25.7128)
  line L8664 (-20.4644, 25.7128) -> (-20.4644, 26.7128)
  line L8665 (-20.4644, 26.7128) -> (-19.4644, 26.7128)
  line L8666 (-19.4644, 26.7128) -> (-19.4644, 25.7128)
  line L8667 (-20.3534, 25.7128) -> (-21.3534, 25.7128)
  line L8668 (-21.3534, 25.7128) -> (-21.3534, 26.7128)
  line L8669 (-21.3534, 26.7128) -> (-20.3534, 26.7128)
  line L8670 (-20.3534, 26.7128) -> (-20.3534, 25.7128)
  line L8671 (-21.1027, 25.7128) -> (-22.1027, 25.7128)
  line L8672 (-22.1027, 25.7128) -> (-22.1027, 26.7128)
  line L8673 (-22.1027, 26.7128) -> (-21.1027, 26.7128)
  line L8674 (-21.1027, 26.7128) -> (-21.1027, 25.7128)
  line L8675 (-21.9663, 25.7128) -> (-22.9663, 25.7128)
  line L8676 (-22.9663, 25.7128) -> (-22.9663, 26.7128)
  line L8677 (-22.9663, 26.7128) -> (-21.9663, 26.7128)
  line L8678 (-21.9663, 26.7128) -> (-21.9663, 25.7128)
  line L8679 (-12.6826, 25.7382) -> (-13.6826, 25.7382)
  line L8680 (-13.6826, 25.7382) -> (-13.6826, 26.7382)
  line L8681 (-13.6826, 26.7382) -> (-12.6826, 26.7382)
  line L8682 (-12.6826, 26.7382) -> (-12.6826, 25.7382)
  line L8683 (-14.4098, 25.7382) -> (-15.4098, 25.7382)
  line L8684 (-15.4098, 25.7382) -> (-15.4098, 26.7382)
  line L8685 (-15.4098, 26.7382) -> (-14.4098, 26.7382)
  line L8686 (-14.4098, 26.7382) -> (-14.4098, 25.7382)
  line L8687 (-14.9813, 25.7382) -> (-15.9813, 25.7382)
  line L8688 (-15.9813, 25.7382) -> (-15.9813, 26.7382)
  line L8689 (-15.9813, 26.7382) -> (-14.9813, 26.7382)
  line L8690 (-14.9813, 26.7382) -> (-14.9813, 25.7382)
  line L8691 (-15.8068, 25.7382) -> (-16.8068, 25.7382)
  line L8692 (-16.8068, 25.7382) -> (-16.8068, 26.7382)
  line L8693 (-16.8068, 26.7382) -> (-15.8068, 26.7382)
  line L8694 (-15.8068, 26.7382) -> (-15.8068, 25.7382)
  line L8695 (-17.1149, 25.7382) -> (-18.1149, 25.7382)
  line L8696 (-18.1149, 25.7382) -> (-18.1149, 26.7382)
  line L8697 (-18.1149, 26.7382) -> (-17.1149, 26.7382)
  line L8698 (-17.1149, 26.7382) -> (-17.1149, 25.7382)
  line L8699 (-18.5246, 25.7382) -> (-19.5246, 25.7382)
  line L8700 (-19.5246, 25.7382) -> (-19.5246, 26.7382)
  line L8701 (-19.5246, 26.7382) -> (-18.5246, 26.7382)
  line L8702 (-18.5246, 26.7382) -> (-18.5246, 25.7382)
  line L8703 (-19.4644, 25.7382) -> (-20.4644, 25.7382)
  line L8704 (-20.4644, 25.7382) -> (-20.4644, 26.7382)
  line L8705 (-20.4644, 26.7382) -> (-19.4644, 26.7382)
  line L8706 (-19.4644, 26.7382) -> (-19.4644, 25.7382)
  line L8707 (-20.3534, 25.7382) -> (-21.3534, 25.7382)
  line L8708 (-21.3534, 25.7382) -> (-21.3534, 26.7382)
  line L8709 (-21.3534, 26.7382) -> (-20.3534, 26.7382)
  line L8710 (-20.3534, 26.7382) -> (-20.3534, 25.7382)
  line L8711 (-21.1027, 25.7382) -> (-22.1027, 25.7382)
  line L8712 (-22.1027, 25.7382) -> (-22.1027, 26.7382)
  line L8713 (-22.1027, 26.7382) -> (-21.1027, 26.7382)
  line L8714 (-21.1027, 26.7382) -> (-21.1027, 25.7382)
  line L8715 (-21.9917, 25.7382) -> (-22.9917, 25.7382)
  line L8716 (-22.9917, 25.7382) -> (-22.9917, 26.7382)
  line L8717 (-22.9917, 26.7382) -> (-21.9917, 26.7382)
  line L8718 (-21.9917, 26.7382) -> (-21.9917, 25.7382)
  line L8719 (-12.708, 25.7636) -> (-13.708, 25.7636)
  line L8720 (-13.708, 25.7636) -> (-13.708, 26.7636)
  line L8721 (-13.708, 26.7636) -> (-12.708, 26.7636)
  line L8722 (-12.708, 26.7636) -> (-12.708, 25.7636)
  line L8723 (-14.4225, 25.7636) -> (-15.4225, 25.7636)
  line L8724 (-15.4225, 25.7636) -> (-15.4225, 26.7636)
  line L8725 (-15.4225, 26.7636) -> (-14.4225, 26.7636)
  line L8726 (-14.4225, 26.7636) -> (-14.4225, 25.7636)
  line L8727 (-15.0067, 25.7636) -> (-16.0067, 25.7636)
  line L8728 (-16.0067, 25.7636) -> (-16.0067, 26.7636)
  line L8729 (-16.0067, 26.7636) -> (-15.0067, 26.7636)
  line L8730 (-15.0067, 26.7636) -> (-15.0067, 25.7636)
  line L8731 (-19.4517, 25.7636) -> (-20.4517, 25.7636)
  line L8732 (-20.4517, 25.7636) -> (-20.4517, 26.7636)
  line L8733 (-20.4517, 26.7636) -> (-19.4517, 26.7636)
  line L8734 (-19.4517, 26.7636) -> (-19.4517, 25.7636)
  line L8735 (-20.3534, 25.7636) -> (-21.3534, 25.7636)
  line L8736 (-21.3534, 25.7636) -> (-21.3534, 26.7636)
  line L8737 (-21.3534, 26.7636) -> (-20.3534, 26.7636)
  line L8738 (-20.3534, 26.7636) -> (-20.3534, 25.7636)
  line L8739 (-21.09, 25.7636) -> (-22.09, 25.7636)
  line L8740 (-22.09, 25.7636) -> (-22.09, 26.7636)
  line L8741 (-22.09, 26.7636) -> (-21.09, 26.7636)
  line L8742 (-21.09, 26.7636) -> (-21.09, 25.7636)
  line L8743 (-21.9917, 25.7636) -> (-22.9917, 25.7636)
  line L8744 (-22.9917, 25.7636) -> (-22.9917, 26.7636)
  line L8745 (-22.9917, 26.7636) -> (-21.9917, 26.7636)
  line L8746 (-21.9917, 26.7636) -> (-21.9917, 25.7636)
  line L8747 (-12.7334, 25.789) -> (-13.7334, 25.789)
  line L8748 (-13.7334, 25.789) -> (-13.7334, 26.789)
  line L8749 (-13.7334, 26.789) -> (-12.7334, 26.789)
  line L8750 (-12.7334, 26.789) -> (-12.7334, 25.789)
  line L8751 (-14.4479, 25.789) -> (-15.4479, 25.789)
  line L8752 (-15.4479, 25.789) -> (-15.4479, 26.789)
  line L8753 (-15.4479, 26.789) -> (-14.4479, 26.789)
  line L8754 (-14.4479, 26.789) -> (-14.4479, 25.789)
  line L8755 (-15.0321, 25.789) -> (-16.0321, 25.789)
  line L8756 (-16.0321, 25.789) -> (-16.0321, 26.789)
  line L8757 (-16.0321, 26.789) -> (-15.0321, 26.789)
  line L8758 (-15.0321, 26.789) -> (-15.0321, 25.789)
  line L8759 (-19.4517, 25.789) -> (-20.4517, 25.789)
  line L8760 (-20.4517, 25.789) -> (-20.4517, 26.789)
  line L8761 (-20.4517, 26.789) -> (-19.4517, 26.789)
  line L8762 (-19.4517, 26.789) -> (-19.4517, 25.789)
  line L8763 (-20.3661, 25.789) -> (-21.3661, 25.789)
  line L8764 (-21.3661, 25.789) -> (-21.3661, 26.789)
  line L8765 (-21.3661, 26.789) -> (-20.3661, 26.789)
  line L8766 (-20.3661, 26.789) -> (-20.3661, 25.789)
  line L8767 (-21.0773, 25.789) -> (-22.0773, 25.789)
  line L8768 (-22.0773, 25.789) -> (-22.0773, 26.789)
  line L8769 (-22.0773, 26.789) -> (-21.0773, 26.789)
  line L8770 (-21.0773, 26.789) -> (-21.0773, 25.789)
  line L8771 (-22.0171, 25.789) -> (-23.0171, 25.789)
  line L8772 (-23.0171, 25.789) -> (-23.0171, 26.789)
  line L8773 (-23.0171, 26.789) -> (-22.0171, 26.789)
  line L8774 (-22.0171, 26.789) -> (-22.0171, 25.789)
  line L8775 (-12.7588, 25.8144) -> (-13.7588, 25.8144)
  line L8776 (-13.7588, 25.8144) -> (-13.7588, 26.8144)
  line L8777 (-13.7588, 26.8144) -> (-12.7588, 26.8144)
  line L8778 (-12.7588, 26.8144) -> (-12.7588, 25.8144)
  line L8779 (-14.4733, 25.8144) -> (-15.4733, 25.8144)
  line L8780 (-15.4733, 25.8144) -> (-15.4733, 26.8144)
  line L8781 (-15.4733, 26.8144) -> (-14.4733, 26.8144)
  line L8782 (-14.4733, 26.8144) -> (-14.4733, 25.8144)
  line L8783 (-19.4517, 25.8144) -> (-20.4517, 25.8144)
  line L8784 (-20.4517, 25.8144) -> (-20.4517, 26.8144)
  line L8785 (-20.4517, 26.8144) -> (-19.4517, 26.8144)
  line L8786 (-19.4517, 26.8144) -> (-19.4517, 25.8144)
  line L8787 (-20.3661, 25.8144) -> (-21.3661, 25.8144)
  line L8788 (-21.3661, 25.8144) -> (-21.3661, 26.8144)
  line L8789 (-21.3661, 26.8144) -> (-20.3661, 26.8144)
  line L8790 (-20.3661, 26.8144) -> (-20.3661, 25.8144)
  line L8791 (-21.0773, 25.8144) -> (-22.0773, 25.8144)
  line L8792 (-22.0773, 25.8144) -> (-22.0773, 26.8144)
  line L8793 (-22.0773, 26.8144) -> (-21.0773, 26.8144)
  line L8794 (-21.0773, 26.8144) -> (-21.0773, 25.8144)
  line L8795 (-22.0171, 25.8144) -> (-23.0171, 25.8144)
  line L8796 (-23.0171, 25.8144) -> (-23.0171, 26.8144)
  line L8797 (-23.0171, 26.8144) -> (-22.0171, 26.8144)
  line L8798 (-22.0171, 26.8144) -> (-22.0171, 25.8144)
  line L8799 (-12.7715, 25.8398) -> (-13.7715, 25.8398)
  line L8800 (-13.7715, 25.8398) -> (-13.7715, 26.8398)
  line L8801 (-13.7715, 26.8398) -> (-12.7715, 26.8398)
  line L8802 (-12.7715, 26.8398) -> (-12.7715, 25.8398)
  line L8803 (-14.4987, 25.8398) -> (-15.4987, 25.8398)
  line L8804 (-15.4987, 25.8398) -> (-15.4987, 26.8398)
  line L8805 (-15.4987, 26.8398) -> (-14.4987, 26.8398)
  line L8806 (-14.4987, 26.8398) -> (-14.4987, 25.8398)
  line L8807 (-19.4517, 25.8398) -> (-20.4517, 25.8398)
  line L8808 (-20.4517, 25.8398) -> (-20.4517, 26.8398)
  line L8809 (-20.4517, 26.8398) -> (-19.4517, 26.8398)
  line L8810 (-19.4517, 26.8398) -> (-19.4517, 25.8398)
  line L8811 (-20.3788, 25.8398) -> (-21.3788, 25.8398)
  line L8812 (-21.3788, 25.8398) -> (-21.3788, 26.8398)
  line L8813 (-21.3788, 26.8398) -> (-20.3788, 26.8398)
  line L8814 (-20.3788, 26.8398) -> (-20.3788, 25.8398)
  line L8815 (-21.0519, 25.8398) -> (-22.0519, 25.8398)
  line L8816 (-22.0519, 25.8398) -> (-22.0519, 26.8398)
  line L8817 (-22.0519, 26.8398) -> (-21.0519, 26.8398)
  line L8818 (-21.0519, 26.8398) -> (-21.0519, 25.8398)
  line L8819 (-22.0425, 25.8398) -> (-23.0425, 25.8398)
  line L8820 (-23.0425, 25.8398) -> (-23.0425, 26.8398)
  line L8821 (-23.0425, 26.8398) -> (-22.0425, 26.8398)
  line L8822 (-22.0425, 26.8398) -> (-22.0425, 25.8398)
  line L8823 (-12.7969, 25.8652) -> (-13.7969, 25.8652)
  line L8824 (-13.7969, 25.8652) -> (-13.7969, 26.8652)
  line L8825 (-13.7969, 26.8652) -> (-12.7969, 26.8652)
  line L8826 (-12.7969, 26.8652) -> (-12.7969, 25.8652)
  line L8827 (-14.5114, 25.8652) -> (-15.5114, 25.8652)
  line L8828 (-15.5114, 25.8652) -> (-15.5114, 26.8652)
  line L8829 (-15.5114, 26.8652) -> (-14.5114, 26.8652)
  line L8830 (-14.5114, 26.8652) -> (-14.5114, 25.8652)
  line L8831 (-19.439, 25.8652) -> (-20.439, 25.8652)
  line L8832 (-20.439, 25.8652) -> (-20.439, 26.8652)
  line L8833 (-20.439, 26.8652) -> (-19.439, 26.8652)
  line L8834 (-19.439, 26.8652) -> (-19.439, 25.8652)
  line L8835 (-20.3788, 25.8652) -> (-21.3788, 25.8652)
  line L8836 (-21.3788, 25.8652) -> (-21.3788, 26.8652)
  line L8837 (-21.3788, 26.8652) -> (-20.3788, 26.8652)
  line L8838 (-20.3788, 26.8652) -> (-20.3788, 25.8652)
  line L8839 (-21.0519, 25.8652) -> (-22.0519, 25.8652)
  line L8840 (-22.0519, 25.8652) -> (-22.0519, 26.8652)
  line L8841 (-22.0519, 26.8652) -> (-21.0519, 26.8652)
  line L8842 (-21.0519, 26.8652) -> (-21.0519, 25.8652)
  line L8843 (-22.0425, 25.8652) -> (-23.0425, 25.8652)
  line L8844 (-23.0425, 25.8652) -> (-23.0425, 26.8652)
  line L8845 (-23.0425, 26.8652) -> (-22.0425, 26.8652)
  line L8846 (-22.0425, 26.8652) -> (-22.0425, 25.8652)
  line L8847 (-12.835, 25.8906) -> (-13.835, 25.8906)
  line L8848 (-13.835, 25.8906) -> (-13.835, 26.8906)
  line L8849 (-13.835, 26.8906) -> (-12.835, 26.8906)
  line L8850 (-12.835, 26.8906) -> (-12.835, 25.8906)
  line L8851 (-14.5368, 25.8906) -> (-15.5368, 25.8906)
  line L8852 (-15.5368, 25.8906) -> (-15.5368, 26.8906)
  line L8853 (-15.5368, 26.8906) -> (-14.5368, 26.8906)
  line L8854 (-14.5368, 26.8906) -> (-14.5368, 25.8906)
  line L8855 (-19.439, 25.8906) -> (-20.439, 25.8906)
  line L8856 (-20.439, 25.8906) -> (-20.439, 26.8906)
  line L8857 (-20.439, 26.8906) -> (-19.439, 26.8906)
  line L8858 (-19.439, 26.8906) -> (-19.439, 25.8906)
  line L8859 (-20.3788, 25.8906) -> (-21.3788, 25.8906)
  line L8860 (-21.3788, 25.8906) -> (-21.3788, 26.8906)
  line L8861 (-21.3788, 26.8906) -> (-20.3788, 26.8906)
  line L8862 (-20.3788, 26.8906) -> (-20.3788, 25.8906)
  line L8863 (-21.0519, 25.8906) -> (-22.0519, 25.8906)
  line L8864 (-22.0519, 25.8906) -> (-22.0519, 26.8906)
  line L8865 (-22.0519, 26.8906) -> (-21.0519, 26.8906)
  line L8866 (-21.0519, 26.8906) -> (-21.0519, 25.8906)
  line L8867 (-22.0679, 25.8906) -> (-23.0679, 25.8906)
  line L8868 (-23.0679, 25.8906) -> (-23.0679, 26.8906)
  line L8869 (-23.0679, 26.8906) -> (-22.0679, 26.8906)
  line L8870 (-22.0679, 26.8906) -> (-22.0679, 25.8906)
  line L8871 (-12.8477, 25.916) -> (-13.8477, 25.916)
  line L8872 (-13.8477, 25.916) -> (-13.8477, 26.916)
  line L8873 (-13.8477, 26.916) -> (-12.8477, 26.916)
  line L8874 (-12.8477, 26.916) -> (-12.8477, 25.916)
  line L8875 (-14.5622, 25.916) -> (-15.5622, 25.916)
  line L8876 (-15.5622, 25.916) -> (-15.5622, 26.916)
  line L8877 (-15.5622, 26.916) -> (-14.5622, 26.916)
  line L8878 (-14.5622, 26.916) -> (-14.5622, 25.916)
  line L8879 (-19.439, 25.916) -> (-20.439, 25.916)
  line L8880 (-20.439, 25.916) -> (-20.439, 26.916)
  line L8881 (-20.439, 26.916) -> (-19.439, 26.916)
  line L8882 (-19.439, 26.916) -> (-19.439, 25.916)
  line L8883 (-20.3915, 25.916) -> (-21.3915, 25.916)
  line L8884 (-21.3915, 25.916) -> (-21.3915, 26.916)
  line L8885 (-21.3915, 26.916) -> (-20.3915, 26.916)
  line L8886 (-20.3915, 26.916) -> (-20.3915, 25.916)
  line L8887 (-21.0392, 25.916) -> (-22.0392, 25.916)
  line L8888 (-22.0392, 25.916) -> (-22.0392, 26.916)
  line L8889 (-22.0392, 26.916) -> (-21.0392, 26.916)
  line L8890 (-21.0392, 26.916) -> (-21.0392, 25.916)
  line L8891 (-22.0679, 25.916) -> (-23.0679, 25.916)
  line L8892 (-23.0679, 25.916) -> (-23.0679, 26.916)
  line L8893 (-23.0679, 26.916) -> (-22.0679, 26.916)
  line L8894 (-22.0679, 26.916) -> (-22.0679, 25.916)
  line L8895 (-12.8731, 25.9414) -> (-13.8731, 25.9414)
  line L8896 (-13.8731, 25.9414) -> (-13.8731, 26.9414)
  line L8897 (-13.8731, 26.9414) -> (-12.8731, 26.9414)
  line L8898 (-12.8731, 26.9414) -> (-12.8731, 25.9414)
  line L8899 (-14.5749, 25.9414) -> (-15.5749, 25.9414)
  line L8900 (-15.5749, 25.9414) -> (-15.5749, 26.9414)
  line L8901 (-15.5749, 26.9414) -> (-14.5749, 26.9414)
  line L8902 (-14.5749, 26.9414) -> (-14.5749, 25.9414)
  line L8903 (-19.4517, 25.9414) -> (-20.4517, 25.9414)
  line L8904 (-20.4517, 25.9414) -> (-20.4517, 26.9414)
  line L8905 (-20.4517, 26.9414) -> (-19.4517, 26.9414)
  line L8906 (-19.4517, 26.9414) -> (-19.4517, 25.9414)
  line L8907 (-20.3915, 25.9414) -> (-21.3915, 25.9414)
  line L8908 (-21.3915, 25.9414) -> (-21.3915, 26.9414)
  line L8909 (-21.3915, 26.9414) -> (-20.3915, 26.9414)
  line L8910 (-20.3915, 26.9414) -> (-20.3915, 25.9414)
  line L8911 (-21.0265, 25.9414) -> (-22.0265, 25.9414)
  line L8912 (-22.0265, 25.9414) -> (-22.0265, 26.9414)
  line L8913 (-22.0265, 26.9414) -> (-21.0265, 26.9414)
  line L8914 (-21.0265, 26.9414) -> (-21.0265, 25.9414)
  line L8915 (-22.0933, 25.9414) -> (-23.0933, 25.9414)
  line L8916 (-23.0933, 25.9414) -> (-23.0933, 26.9414)
  line L8917 (-23.0933, 26.9414) -> (-22.0933, 26.9414)
  line L8918 (-22.0933, 26.9414) -> (-22.0933, 25.9414)
  line L8919 (-12.8985, 25.9668) -> (-13.8985, 25.9668)
  line L8920 (-13.8985, 25.9668) -> (-13.8985, 26.9668)
  line L8921 (-13.8985, 26.9668) -> (-12.8985, 26.9668)
  line L8922 (-12.8985, 26.9668) -> (-12.8985, 25.9668)
  line L8923 (-14.6003, 25.9668) -> (-15.6003, 25.9668)
  line L8924 (-15.6003, 25.9668) -> (-15.6003, 26.9668)
  line L8925 (-15.6003, 26.9668) -> (-14.6003, 26.9668)
  line L8926 (-14.6003, 26.9668) -> (-14.6003, 25.9668)
  line L8927 (-19.439, 25.9668) -> (-20.439, 25.9668)
  line L8928 (-20.439, 25.9668) -> (-20.439, 26.9668)
  line L8929 (-20.439, 26.9668) -> (-19.439, 26.9668)
  line L8930 (-19.439, 26.9668) -> (-19.439, 25.9668)
  line L8931 (-20.3915, 25.9668) -> (-21.3915, 25.9668)
  line L8932 (-21.3915, 25.9668) -> (-21.3915, 26.9668)
  line L8933 (-21.3915, 26.9668) -> (-20.3915, 26.9668)
  line L8934 (-20.3915, 26.9668) -> (-20.3915, 25.9668)
  line L8935 (-21.0265, 25.9668) -> (-22.0265, 25.9668)
  line L8936 (-22.0265, 25.9668) -> (-22.0265, 26.9668)
  line L8937 (-22.0265, 26.9668) -> (-21.0265, 26.9668)
  line L8938 (-21.0265, 26.9668) -> (-21.0265, 25.9668)
  line L8939 (-22.0933, 25.9668) -> (-23.0933, 25.9668)
  line L8940 (-23.0933, 25.9668) -> (-23.0933, 26.9668)
  line L8941 (-23.0933, 26.9668) -> (-22.0933, 26.9668)
  line L8942 (-22.0933, 26.9668) -> (-22.0933, 25.9668)
  line L8943 (-12.9366, 25.9922) -> (-13.9366, 25.9922)
  line L8944 (-13.9366, 25.9922) -> (-13.9366, 26.9922)
  line L8945 (-13.9366, 26.9922) -> (-12.9366, 26.9922)
  line L8946 (-12.9366, 26.9922) -> (-12.9366, 25.9922)
  line L8947 (-14.6257, 25.9922) -> (-15.6257, 25.9922)
  line L8948 (-15.6257, 25.9922) -> (-15.6257, 26.9922)
  line L8949 (-15.6257, 26.9922) -> (-14.6257, 26.9922)
  line L8950 (-14.6257, 26.9922) -> (-14.6257, 25.9922)
  line L8951 (-19.439, 25.9922) -> (-20.439, 25.9922)
  line L8952 (-20.439, 25.9922) -> (-20.439, 26.9922)
  line L8953 (-20.439, 26.9922) -> (-19.439, 26.9922)
  line L8954 (-19.439, 26.9922) -> (-19.439, 25.9922)
  line L8955 (-20.4042, 25.9922) -> (-21.4042, 25.9922)
  line L8956 (-21.4042, 25.9922) -> (-21.4042, 26.9922)
  line L8957 (-21.4042, 26.9922) -> (-20.4042, 26.9922)
  line L8958 (-20.4042, 26.9922) -> (-20.4042, 25.9922)
  line L8959 (-21.0138, 25.9922) -> (-22.0138, 25.9922)
  line L8960 (-22.0138, 25.9922) -> (-22.0138, 26.9922)
  line L8961 (-22.0138, 26.9922) -> (-21.0138, 26.9922)
  line L8962 (-21.0138, 26.9922) -> (-21.0138, 25.9922)
  line L8963 (-22.106, 25.9922) -> (-23.106, 25.9922)
  line L8964 (-23.106, 25.9922) -> (-23.106, 26.9922)
  line L8965 (-23.106, 26.9922) -> (-22.106, 26.9922)
  line L8966 (-22.106, 26.9922) -> (-22.106, 25.9922)
  line L8967 (-12.9493, 26.0176) -> (-13.9493, 26.0176)
  line L8968 (-13.9493, 26.0176) -> (-13.9493, 27.0176)
  line L8969 (-13.9493, 27.0176) -> (-12.9493, 27.0176)
  line L8970 (-12.9493, 27.0176) -> (-12.9493, 26.0176)
  line L8971 (-14.6257, 26.0176) -> (-15.6257, 26.0176)
  line L8972 (-15.6257, 26.0176) -> (-15.6257, 27.0176)
  line L8973 (-15.6257, 27.0176) -> (-14.6257, 27.0176)
  line L8974 (-14.6257, 27.0176) -> (-14.6257, 26.0176)
  line L8975 (-19.439, 26.0176) -> (-20.439, 26.0176)